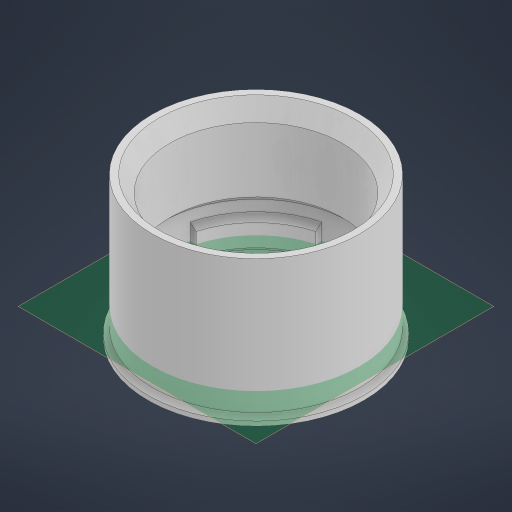
# Autodesk Inventor part: screw_grip
Saved by Autodesk Inventor 2024 (Build 280153000, 153)
## iProperties
Created: 2024-10-06
Part Number: screw_grip
Material: Generic
Document SubType Name: Modeling
Designer: loren
Density: 1 g/cm^3
Appearance: Default
Author: loren
Autodesk Inventor part; units mm, degrees
ref_plane "YZ Plane" through (0, 0, 0) normal (1, 0, 0) x (0, 1, 0)
ref_plane "XZ Plane" through (0, 0, 0) normal (0, 1, 0) x (-1, 0, 0)
ref_plane "XY Plane" through (0, 0, 0) normal (0, 0, 1) x (1, 0, 0)
sketch "Sketch1" plane through (0, 0, 0) normal (0, 1, 0) x (-1, 0, 0)
  line L0 (0, 0) -> (0, 13)
  line L1 (-8.9, 13) -> (-7.9, 11.5)
  line L2 (-7.9, 11.5) -> (-7.9, 5.6)
  line L3 (-7.9, 5.6) -> (-8.5, 5)
  line L4 (-8.5, 5) -> (-8.5, 0)
  line L5 (-8.5, 0) -> (-9.5, 0)
  line L6 (-9.5, 0) -> (-9.5, 13)
  line L7 (-9.5, 13) -> (-8.9, 13)
  line L8 (-9.5, 0.8) -> (-9.9, 0.4)
  line L9 (-9.9, 0.4) -> (-9.9, 0)
  line L10 (-9.9, 0) -> (-9.5, 0)
  dimension "d0" = 15.8
  dimension "d1" = 5
  dimension "d2" = 19
  dimension "d3" = 1
  dimension "d4" = 1.5
  dimension "d5" = 8
  dimension "d6" = 17
  dimension "d7" = 45
  dimension "d9" = 0.8
  dimension "d10" = 0.4
  dimension "d11" = 0.4
  constraints: 22 end point, 3 perpendicular, 3 point on line, 3 vertical, 1 parallel
  measures "d0" diameter of L2 L0
  measures "d1" distance of L3.end L4.end
  measures "d2" diameter of L6 L0
  measures "d3" distance from line of L1.start L2
  measures "d4" vertical distance of L1.start L1.end
  measures "d5" distance from line of L7 L3.end
  measures "d6" diameter of L4 L0
  measures "d7" angle of L2 L3
  measures "d9" distance from line of L10 L8.start
  measures "d10" distance of L8.end L9.end
  measures "d11" distance of L9.end L5.end
revolve "Revolution1" add sketch "Sketch1" angle 360 about axis through (0, 0, 0) along (0, 0, 1)
ref_plane "Work Plane1" through (0, 0, 2.5) normal (0, 0, -1) x (-1, 0, 0)
sketch "Sketch2" plane through (0, 0, 2.5) normal (0, 0, -1) x (-1, 0, 0)
  circle A0 centre (0, 0) radius 8.5 projected
  line L0 (-2.2, 8.2104) -> (-2.2, 7.6916)
  arc A1 (-2.2, 7.6916) -> (-7.6916, 2.2) centre (0, 0) ccw
  line L1 (-7.6916, 2.2) -> (-8.2104, 2.2)
  dimension "d14" = 60
  dimension "d15" = 0.5
  constraints: 4 end point, 4 point on circle, 1 centre point, 1 coincident, 1 horizontal, 1 perpendicular, 1 vertical
  measures "d15" radial gap between concentric circles of A0 A1
extrude "Extrusion1" add sketch "Sketch2" along normal mid plane 3 contours L0 A1 L1 A0 picked at (-5.6701, 6.0517)
chamfer "Chamfer1" distance 0.5 angle 45 2 edges at (5.6569, 5.6569, 4) (5.6569, 5.6569, 1)
pattern_circular "Circular Pattern1" count 4 over 360 about axis through (0, 0, -10) along (0, 0, 1) of "Extrusion1", "Chamfer1"
body "Solid1"
